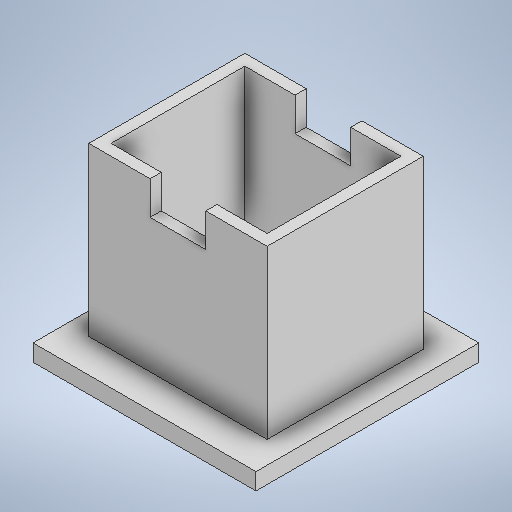
# Autodesk Inventor part: 差分線圈激勵
Saved by Autodesk Inventor 2025.2 (Build 292293000, 293)
## iProperties
Created: 2025-07-14
Part Number: 差分線圈激勵
Material: 一般
Document SubType Name: Modeling
Designer: 123
Density: 1 g/cm^3
Appearance: 預設
Author: 123
Autodesk Inventor part; units mm, degrees
ref_plane "YZ Plane" through (0, 0, 0) normal (1, 0, 0) x (0, 1, 0)
ref_plane "XZ Plane" through (0, 0, 0) normal (0, 1, 0) x (-1, 0, 0)
ref_plane "XY Plane" through (0, 0, 0) normal (0, 0, 1) x (1, 0, 0)
sketch "草圖8" plane through (0, 0, 0) normal (0, 1, 0) x (-1, 0, 0)
  line L0 (10, 10) -> (-10, 10)
  line L1 (-10, 10) -> (-10, -10)
  line L2 (-10, -10) -> (10, -10)
  line L3 (10, -10) -> (10, 10)
  line L4 (10, 10) -> (-10, -10) construction
  line L5 (-10, 10) -> (10, -10) construction
  point P0 (0, 0)
  dimension "d36" = 20
  dimension "d37" = 20
  constraints: 12 end point, 2 midpoint, 2 parallel, 1 horizontal, 1 perpendicular
  measures "d36" distance of L1.end L2.end
  measures "d37" distance of L2.end L0.start
extrude "擠出8" add sketch "草圖8" along normal blind 1.5
sketch "草圖9" plane through (0, 1.5, 0) normal (0, 1, 0) x (1, 0, 0)
  line L0 (-8, -7) -> (8, -7)
  line L1 (8, -7) -> (8, 7)
  line L2 (8, 7) -> (-8, 7)
  line L3 (-8, 7) -> (-8, -7)
  line L4 (-8, -7) -> (8, 7) construction
  line L5 (8, -7) -> (-8, 7) construction
  line L6 (-7, 6) -> (7, 6)
  line L7 (7, 6) -> (7, -6)
  line L8 (7, -6) -> (-7, -6)
  line L9 (-7, -6) -> (-7, 6)
  line L10 (-7, 6) -> (7, -6) construction
  line L11 (7, 6) -> (-7, -6) construction
  point P0 (0, 0)
  dimension "d40" = 16
  dimension "d41" = 14
  dimension "d46" = 14
  dimension "d47" = 12
  constraints: 24 end point, 4 midpoint, 4 parallel, 2 horizontal, 2 perpendicular
  measures "d40" distance of L1.end L2.end
  measures "d41" distance of L2.end L0.start
  measures "d46" distance of L6.start L6.end
  measures "d47" distance of L8.end L6.start
extrude "擠出10" add sketch "草圖9" along normal blind 15
sketch "草圖11" plane through (-8, 1.5, 7) normal (0, 0, 1) x (1, 0, 0)
  line L0 (5.5, 18) -> (10.5, 18)
  line L1 (10.5, 18) -> (10.5, 12)
  line L2 (10.5, 12) -> (5.5, 12)
  line L3 (5.5, 12) -> (5.5, 18)
  line L4 (16, 15) -> (0, 15) projected
  line L5 (5.5, 18) -> (10.5, 12) construction
  line L6 (10.5, 18) -> (5.5, 12) construction
  point P0 (8, -1.5)
  point P1 (8, 15)
  point P2 (10.5, 15)
  point P3 (5.5, 15)
  dimension "d50" = 5
  dimension "d51" = 6
  constraints: 12 end point, 3 midpoint, 2 parallel, 1 horizontal, 1 perpendicular
  measures "d50" distance of L1.end L2.end
  measures "d51" distance of L0.end L1.end
extrude "擠出11" cut sketch "草圖11" against normal blind 15 contours L4 L1 L2 L3
sketch "草圖12" plane through (0, 1.5, 0) normal (0, 1, 0) x (1, 0, 0)
  line L0 (-4.5, 2.5) -> (-2.5, 2.5)
  line L1 (-2.5, 2.5) -> (-2.5, -2.5)
  line L2 (-2.5, -2.5) -> (-4.5, -2.5)
  line L3 (-4.5, -2.5) -> (-4.5, 2.5)
  line L4 (-4.5, 2.5) -> (-2.5, -2.5) construction
  line L5 (-2.5, 2.5) -> (-4.5, -2.5) construction
  line L6 (2.5, 2.5) -> (4.5, 2.5)
  line L7 (4.5, 2.5) -> (4.5, -2.5)
  line L8 (4.5, -2.5) -> (2.5, -2.5)
  line L9 (2.5, -2.5) -> (2.5, 2.5)
  line L10 (2.5, 2.5) -> (4.5, -2.5) construction
  line L11 (4.5, 2.5) -> (2.5, -2.5) construction
  line L12 (7, 6) -> (7, -6) projected
  point P0 (0, 0)
  point P1 (-3.5, 0)
  point P2 (3.5, 0)
  point P3 (7, 0)
  dimension "d54" = 5
  dimension "d55" = 2
  dimension "d56" = 5
  dimension "d57" = 2
  dimension "d58" = 3.5
  dimension "d59" = 3.5
  dimension "d60" = 3.5
  constraints: 24 end point, 5 midpoint, 4 parallel, 2 horizontal, 2 perpendicular, 1 point on line
  measures "d54" distance of L0.end L1.end
  measures "d55" distance of L0.start L0.end
  measures "d56" distance of L8.end L6.start
  measures "d57" distance of L6.start L6.end
  measures "d58" distance of point (0, 0) point (-3.5, 0)
  measures "d59" distance of point (0, 0) point (3.5, 0)
  measures "d60" distance of point (7, 0) point (3.5, 0)
extrude "擠出12" add sketch "草圖12" along normal blind 1
